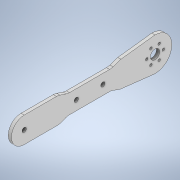
# Autodesk Inventor part: Brazo1.1
Saved by Autodesk Inventor 2022 (Build 260153000, 153)
## iProperties
Created: 2021-09-09
Part Number: Brazo1.1
Material: Generic
Document SubType Name: Modeling
Designer: Administrador
Density: 1 g/cm^3
Appearance: Default
Author: Administrador
Autodesk Inventor part; units mm, degrees
ref_plane "YZ Plane" through (0, 0, 0) normal (1, 0, 0) x (0, 1, 0)
ref_plane "XZ Plane" through (0, 0, 0) normal (0, 1, 0) x (-1, 0, 0)
ref_plane "XY Plane" through (0, 0, 0) normal (0, 0, 1) x (1, 0, 0)
sketch "Sketch1" plane through (0, 0, 0) normal (1, 0, 0) x (0, 1, 0)
  circle A0 centre (12, -104.7) radius 4.375
  circle A1 centre (12, -104.7) radius 9 construction
  line L0 (12, -116.7) -> (12, -104.7) construction
  line L1 (12, -113.7) -> (12, -112.5)
  circle A2 centre (12, -112.5) radius 1.2
  circle A3 centre (12, -55.7) radius 2
  circle A4 centre (18.755, -108.6) radius 1.2
  circle A5 centre (18.755, -100.8) radius 1.2
  circle A6 centre (12, -96.9) radius 1.2
  circle A7 centre (5.245, -100.8) radius 1.2
  circle A8 centre (5.245, -108.6) radius 1.2
  line L2 (3, -43.2) -> (21, -43.2) construction
  line L3 (12, -116.7) -> (12, -71.7) construction
  line L4 (12, -71.7) -> (12, -63.7) construction
  line L5 (12, -63.7) -> (21, -63.7) construction
  line L6 (12, -63.7) -> (3, -63.7) construction
  line L7 (24, -72.7) -> (21, -63.7)
  line L8 (0, -71.7) -> (3, -63.7)
  line L9 (3, -43.2) -> (3, -63.7)
  line L10 (21, -43.2) -> (21, -63.7)
  arc A9 (24, 18.3) -> (0, 18.3) centre (12, 18.3) ccw
  circle A10 centre (12, -30.7) radius 2
  line L11 (12, -14.7) -> (12, -22.7) construction
  line L12 (12, -22.7) -> (21, -22.7) construction
  line L13 (12, -22.7) -> (3, -22.7) construction
  line L14 (24, -13.7) -> (21, -22.7)
  line L15 (0, -14.7) -> (3, -22.7)
  line L16 (3, -43.2) -> (3, -22.7)
  line L17 (0, 18.3) -> (0, -14.7)
  line L18 (24, 18.3) -> (24, -13.7)
  line L19 (21, -43.2) -> (21, -22.7)
  arc A11 (-3.3865, -101.1088) -> (27.3606, -100.9997) centre (12, -104.7) ccw
  line L20 (24, -72.7) -> (27.8, -104.7)
  line L21 (0, -71.7) -> (-3.8, -104.7)
  circle A12 centre (12, 18.3) radius 2
  point P0 (1.5, 26.1095)
  point P1 (22.5, 26.1095)
  point P2 (19.7942, -109.2)
  point P3 (19.7942, -100.2)
  point P4 (12, -95.7)
  point P5 (4.2058, -100.2)
  point P6 (4.2058, -109.2)
  dimension "d7" = 18
  dimension "d6" = 8.75
  dimension "d8" = 1.2
  dimension "d12" = 4
  dimension "d15" = 360
  dimension "d22" = 45
  dimension "d23" = 8
  dimension "d24" = 9
  dimension "d25" = 9
  dimension "d33" = 8
  dimension "d34" = 12.5
  dimension "d45" = 4
  dimension "d46" = 4
  constraints: 44 end point, 7 symmetric about line, 6 centre point, 6 point on circle, 4 point on line, 4 vertical, 3 coincident, 3 horizontal, 3 vertical alignment, 1 perpendicular, 38 other
  measures "d6" diameter of A0
  measures "d8" distance of L1.start L1.end
  measures "d12" diameter of A3
  measures "d22" distance of L0.start L3.end
  measures "d23" distance of L3.end L4.end
  measures "d24" distance of L4.end L5.end
  measures "d25" distance of L4.end L6.end
  measures "d33" distance of A3.centre L4.end
  measures "d34" distance from line of L2 A3.centre
  measures "d45" diameter of A12
  measures "d46" diameter of A10
extrude "Extrusion2" add sketch "Sketch1" along normal blind 3 contours L20 A11 L21 L8 L9 L16 L15 L17 A9 L18 L14 L19 L10 L7
fillet "Face Fillet1" radius 10 1 edges at (1.5, 3, -22.7)
fillet "Face Fillet2" radius 10 1 edges at (1.5, 0, -14.7)
fillet "Face Fillet3" radius 10 1 edges at (1.5, 3, -63.7)
fillet "Face Fillet5" radius 10 1 edges at (1.5, 24, -13.7)
fillet "Face Fillet6" radius 10 1 edges at (1.5, 21, -22.7)
fillet "Face Fillet7" radius 10 1 edges at (1.5, 21, -63.7)
body "Solid2"
